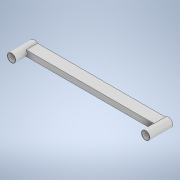
# Autodesk Inventor part: bocina1
Saved by Autodesk Inventor 2021 (Build 250183000, 183)
## iProperties
Created: 2022-01-26
Part Number: bocina1
Material: Genérico
Document SubType Name: Modeling
Designer: arthu
Density: 1 g/cm^3
Appearance: Valor por defecto
Author: arthu
Autodesk Inventor part; units mm, degrees
ref_plane "YZ Plane" through (0, 0, 0) normal (1, 0, 0) x (0, 1, 0)
ref_plane "XZ Plane" through (0, 0, 0) normal (0, 1, 0) x (-1, 0, 0)
ref_plane "XY Plane" through (0, 0, 0) normal (0, 0, 1) x (1, 0, 0)
sketch "Boceto1" plane through (0, 0, 0) normal (0, 0, 1) x (1, 0, 0)
  circle A0 centre (0, 0) radius 30
  circle A1 centre (0, 0) radius 26.15
  circle A2 centre (940, 0) radius 30
  circle A3 centre (940, 0) radius 26.15
  line L0 (22.3607, -20) -> (917.6393, -20)
  line L1 (26.15, 0) -> (30, 0)
  line L2 (910, 0) -> (940, 0)
  line L3 (22.3607, 20) -> (917.6393, 20)
  dimension "d1" = 52.3
  dimension "d0" = 60
  dimension "d2" = 940
  dimension "d3" = 60
  dimension "d4" = 52.3
  constraints: 8 end point, 6 point on circle, 4 coincident, 4 parallel, 3 centre point, 2 horizontal, 1 horizontal alignment, 2 other
  measures "d0" diameter of A0
  measures "d2" distance of point (0, 0) L2.end
  measures "d3" diameter of A2
  measures "d4" diameter of A3
extrude "Extrusión1" add sketch "Boceto1" along normal blind 80
sketch "Boceto2" plane through (0, 0, 80) normal (0, 0, 1) x (1, 0, 0)
  arc A0 (22.3607, 20) -> (22.3607, -20) centre (0, 0) ccw projected
  line L0 (22.3607, -20) -> (917.6393, -20) projected
  arc A1 (917.6393, -20) -> (917.6393, 20) centre (940, 0) ccw projected
  line L1 (917.6393, 20) -> (22.3607, 20) projected
  circle A2 centre (0, 0) radius 26.15 projected
  circle A3 centre (940, 0) radius 26.15 projected
  line L2 (917.6393, 20) -> (22.3607, 20) projected
  circle A4 centre (0, 0) radius 30
  circle A5 centre (940, 0) radius 30
  point P0 (22.3607, -20)
  constraints: 2 coincident, 6 other
extrude "Extrusión2" add sketch "Boceto2" along normal blind 80 contours A4 A0 | A1 A5
